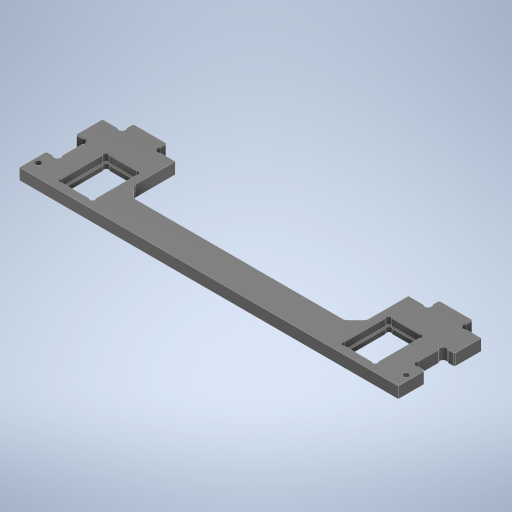
# Autodesk Inventor part: TorsoElectronicBoxUpperFrame
Saved by Autodesk Inventor 2024.2 (Build 282272000, 272)
## iProperties
Created: 2024-01-24
Part Number: TorsoElectronicBoxUpperFrame
Material: Acetal Resin, Black
Document SubType Name: Modeling
Designer: Masato Kubotera
Density: 1.425 g/cm^3
Appearance: Smooth - Black
Mass: 23.1569 g
Surface Area: 99.1055 cm^2
Volume: 16.2504 cm^3
Vendor: meviy
Author: Masato Kubotera
Autodesk Inventor part; units mm, degrees
ref_plane "YZ Plane" through (0, 0, 0) normal (1, 0, 0) x (0, 1, 0)
ref_plane "XZ Plane" through (0, 0, 0) normal (0, 1, 0) x (-1, 0, 0)
ref_plane "XY Plane" through (0, 0, 0) normal (0, 0, 1) x (1, 0, 0)
sketch "Sketch1" plane through (0, 0, 0) normal (0, 0, 1) x (1, 0, 0)
  line L0 (0, -84.5) -> (0, -75.75)
  line L1 (0, -75.75) -> (-5, -75.75)
  line L2 (-5, -75.75) -> (-5, -60.75)
  line L3 (-5, -60.75) -> (0, -60.75)
  line L4 (0, -60.75) -> (0, 60.75)
  line L5 (0, 0) -> (37, 0) construction
  line L6 (0, -84.5) -> (11.95, -84.5)
  line L7 (11.95, -84.5) -> (11.95, -79.5)
  line L8 (11.95, -79.5) -> (25.05, -79.5)
  line L9 (25.05, -79.5) -> (25.05, -84.5)
  line L10 (25.05, -84.5) -> (37, -84.5)
  line L11 (37, -84.5) -> (37, 84.5)
  line L12 (0, 84.5) -> (0, 75.75)
  line L13 (0, 75.75) -> (-5, 75.75)
  line L14 (-5, 75.75) -> (-5, 60.75)
  line L15 (-5, 60.75) -> (0, 60.75)
  line L16 (0, 84.5) -> (11.95, 84.5)
  line L17 (11.95, 84.5) -> (11.95, 79.5)
  line L18 (11.95, 79.5) -> (25.05, 79.5)
  line L19 (25.05, 79.5) -> (25.05, 84.5)
  line L20 (25.05, 84.5) -> (37, 84.5)
  arc A0 (14.0713, -79.5) -> (11.95, -81.6213) centre (13.0107, -80.5607) ccw
  line L21 (12, -84.5) -> (12, -79.5) construction
  line L22 (18.5, -79.5) -> (18.5, -84.5) construction
  line L23 (25, -84.5) -> (25, -79.5) construction
  arc A1 (0, -77.8713) -> (-2.1213, -75.75) centre (-1.0607, -76.8107) ccw
  line L24 (-5, -68.25) -> (0, -68.25) construction
  arc A2 (-2.1213, -60.75) -> (0, -58.6287) centre (-1.0607, -59.6893) ccw
  arc A3 (25.05, -81.6213) -> (22.9287, -79.5) centre (23.9893, -80.5607) ccw
  line L25 (18.5, -82) -> (31, -82) construction
  arc A4 (11.95, 81.6213) -> (14.0713, 79.5) centre (13.0107, 80.5607) ccw
  arc A5 (-2.1213, 75.75) -> (0, 77.8713) centre (-1.0607, 76.8107) ccw
  arc A6 (0, 58.6287) -> (-2.1213, 60.75) centre (-1.0607, 59.6893) ccw
  arc A7 (22.9287, 79.5) -> (25.05, 81.6213) centre (23.9893, 80.5607) ccw
  line L26 (0, -52) -> (23.5, -52)
  line L27 (23.5, -52) -> (23.5, 52)
  line L28 (23.5, 52) -> (0, 52)
  line L29 (23, 51.5) -> (23, -51.5) construction
  line L30 (32.5, -69.5) -> (13.3, -69.5) construction
  line L31 (13.3, -69.5) -> (13.3, -56.6) construction
  line L32 (13.3, -56.6) -> (32.5, -56.6) construction
  line L33 (32.5, -56.6) -> (32.5, -69.5) construction
  line L34 (32.5, -69.5) -> (13.3, -56.6) construction
  line L35 (13.3, -69.5) -> (32.5, -56.6) construction
  line L36 (12.35, -55.5) -> (33.45, -55.5) construction
  line L37 (33.45, -55.5) -> (33.45, -70.6) construction
  line L38 (33.45, -70.6) -> (12.35, -70.6) construction
  line L39 (12.35, -70.6) -> (12.35, -55.5) construction
  line L40 (12.35, -55.5) -> (33.45, -70.6) construction
  line L41 (33.45, -55.5) -> (12.35, -70.6) construction
  line L42 (13.7849, -55.45) -> (32.0151, -55.45)
  line L43 (33.5, -56.9349) -> (33.5, -69.1651)
  line L44 (33.5, -70.65) -> (12.3, -55.45) construction
  line L45 (12.3, -70.65) -> (33.5, -55.45) construction
  line L46 (32.55, -69.55) -> (13.25, -56.55) construction
  line L47 (13.25, -69.55) -> (32.55, -56.55) construction
  arc A8 (13.7849, -55.45) -> (12.3, -56.9349) centre (13.0425, -56.1925) ccw
  arc A9 (14.7349, -56.55) -> (13.25, -58.0349) centre (13.9925, -57.2925) ccw
  line L48 (12.3, -63.05) -> (33.5, -63.05) construction
  line L49 (22.9, -55.45) -> (22.9, -70.65) construction
  arc A10 (33.5, -56.9349) -> (32.0151, -55.45) centre (32.7575, -56.1925) ccw
  arc A11 (32.55, -58.0349) -> (31.0651, -56.55) centre (31.8075, -57.2925) ccw
  arc A12 (13.25, -68.0651) -> (14.7349, -69.55) centre (13.9925, -68.8075) ccw
  arc A13 (12.3, -69.1651) -> (13.7849, -70.65) centre (13.0425, -69.9075) ccw
  arc A14 (31.0651, -69.55) -> (32.55, -68.0651) centre (31.8075, -68.8075) ccw
  arc A15 (32.0151, -70.65) -> (33.5, -69.1651) centre (32.7575, -69.9075) ccw
  line L50 (14.7349, -56.55) -> (31.0651, -56.55)
  line L51 (32.55, -58.0349) -> (32.55, -68.0651)
  line L52 (12.3, -69.1651) -> (12.3, -56.9349)
  line L53 (13.25, -68.0651) -> (13.25, -58.0349)
  line L54 (31.0651, -69.55) -> (14.7349, -69.55)
  line L55 (32.0151, -70.65) -> (13.7849, -70.65)
  line L56 (13.3, 69.5) -> (13.3, 56.6) construction
  arc A16 (12.3, 56.9349) -> (13.7849, 55.45) centre (13.0425, 56.1925) ccw
  arc A17 (13.7849, 70.65) -> (12.3, 69.1651) centre (13.0425, 69.9075) ccw
  line L57 (14.7349, 56.55) -> (31.0651, 56.55)
  arc A18 (32.0151, 55.45) -> (33.5, 56.9349) centre (32.7575, 56.1925) ccw
  arc A19 (31.0651, 56.55) -> (32.55, 58.0349) centre (31.8075, 57.2925) ccw
  line L58 (32.55, 58.0349) -> (32.55, 68.0651)
  line L59 (33.5, 56.9349) -> (33.5, 69.1651)
  line L60 (31.0651, 69.55) -> (14.7349, 69.55)
  arc A20 (32.55, 68.0651) -> (31.0651, 69.55) centre (31.8075, 68.8075) ccw
  arc A21 (33.5, 69.1651) -> (32.0151, 70.65) centre (32.7575, 69.9075) ccw
  line L61 (32.0151, 70.65) -> (13.7849, 70.65)
  line L62 (22.9, 55.45) -> (22.9, 70.65) construction
  line L63 (13.7849, 55.45) -> (32.0151, 55.45)
  line L64 (32.5, 69.5) -> (13.3, 69.5) construction
  line L65 (13.3, 56.6) -> (32.5, 56.6) construction
  line L66 (32.5, 56.6) -> (32.5, 69.5) construction
  line L67 (32.5, 69.5) -> (13.3, 56.6) construction
  line L68 (13.3, 69.5) -> (32.5, 56.6) construction
  line L69 (12.35, 55.5) -> (33.45, 55.5) construction
  line L70 (33.45, 55.5) -> (33.45, 70.6) construction
  line L71 (33.45, 70.6) -> (12.35, 70.6) construction
  line L72 (12.35, 70.6) -> (12.35, 55.5) construction
  line L73 (12.35, 55.5) -> (33.45, 70.6) construction
  line L74 (33.45, 55.5) -> (12.35, 70.6) construction
  line L75 (12.3, 70.65) -> (33.5, 55.45) construction
  line L76 (32.55, 69.55) -> (13.25, 56.55) construction
  line L77 (13.25, 69.55) -> (32.55, 56.55) construction
  arc A22 (13.25, 58.0349) -> (14.7349, 56.55) centre (13.9925, 57.2925) ccw
  line L78 (12.3, 63.05) -> (33.5, 63.05) construction
  arc A23 (14.7349, 69.55) -> (13.25, 68.0651) centre (13.9925, 68.8075) ccw
  line L79 (13.25, 68.0651) -> (13.25, 58.0349)
  line L80 (12.3, 69.1651) -> (12.3, 56.9349)
  line L81 (33.5, 70.65) -> (12.3, 55.45) construction
  line L82 (23, -51.5) -> (0, -51.5) construction
  line L83 (23, 51.5) -> (0, 51.5) construction
  point P0 (31, 82)
  point P1 (22.9287, -79.5)
  point P2 (25.05, -81.6213)
  point P3 (25.05, 81.6213)
  point P4 (22.9287, 79.5)
  point P5 (14.0713, 79.5)
  point P6 (11.95, 81.6213)
  point P7 (0, 77.8713)
  point P8 (-2.1213, 75.75)
  point P9 (-2.1213, 60.75)
  point P10 (0, 58.6287)
  point P11 (0, -58.6287)
  point P12 (-2.1213, -60.75)
  point P13 (22.9, -63.05)
  point P14 (22.9, -63.05)
  point P15 (22.9, 63.05)
  point P16 (22.9, 63.05)
  point P17 (25.05, 79.5)
  point P18 (0, 60.75)
  point P19 (25.05, 79.5)
  point P20 (0, 75.75)
  point P21 (0, 60.75)
  point P22 (11.95, 79.5)
  point P23 (0, 75.75)
  point P24 (11.95, 79.5)
  point P25 (0, -60.75)
  point P26 (25.05, -79.5)
  point P27 (0, -60.75)
  point P28 (0, -52)
  dimension "d0" = 5
  dimension "d1" = 5
  dimension "d2" = 1.5
  dimension "d4" = 15
  dimension "d5" = 0.05
  dimension "d6" = 12
  dimension "d7" = 169
  dimension "d8" = 37
  dimension "d9" = 6
  dimension "d22" = 23
  dimension "d28" = 19.2
  dimension "d29" = 12.9
  dimension "d30" = 21.1
  dimension "d31" = 15.1
  dimension "d32" = 0.05
  dimension "d33" = 1.05
  dimension "d34" = 1.05
  dimension "d35" = 0.05
  dimension "d36" = 0.05
  dimension "d37" = 0.05
  dimension "d44" = 3.5
  dimension "d46" = 3.5
  dimension "d52" = 13.5
  dimension "d53" = 0.5
  dimension "d54" = 103
  dimension "d55" = 0.5
  dimension "d60" = 22.5
  constraints: 168 end point, 96 symmetric about line, 58 point on circle, 29 midpoint, 27 point on line, 24 centre point, 13 horizontal, 9 parallel, 7 vertical, 6 perpendicular, 1 equal radius, 23 other
  measures "d0" distance of L0.end L1.end
  measures "d1" distance of L7.end L6.end
  measures "d2" radius of A0
  measures "d4" distance of L1.end L2.end
  measures "d5" distance between parallel lines of L21 L7
  measures "d6" distance between parallel lines of L21 L0
  measures "d7" distance of L10.end L11.end
  measures "d8" distance of L10.end L0.start
  measures "d9" distance from line of L25.end L23
  measures "d22" distance between parallel lines of L4 L29
  measures "d28" distance of L31.end L32.end
  measures "d29" distance of L31.start L31.end
  measures "d30" distance of L37.end L38.end
  measures "d31" distance of L36.end L37.end
  measures "d32" distance between parallel lines of L42 L36
  measures "d33" radius of A8
  measures "d34" radius of A9
  measures "d35" distance between parallel lines of L50 L32
  measures "d36" distance between parallel lines of L52 L39
  measures "d37" distance between parallel lines of L53 L31
  measures "d44" distance between parallel lines of L11 L43
  measures "d46" distance between parallel lines of L26 L36
  measures "d52" distance between parallel lines of L11 L27
  measures "d53" distance between parallel lines of L27 L29
  measures "d54" distance of L29.start L29.end
  measures "d55" distance between parallel lines of L82 L26
  measures "d60" diameter of L8 L24
extrude "Extrusion1" add sketch "Sketch1" against normal blind 5 contours L0 A1 L1 L2 L3 A2 L4 L26 L27 L28 A6 L15 L14 L13 A5 L12 L16 L17 A4 L18 A7 L19 L20 L11 L10 L9 A3 L8 A0 L7 L6 | L42 A10 L43 A15 L55 A13 L52 A8 | L80 A17 L61 A21 L59 A18 L63 A16
extrude "Extrusion2" cut sketch "Sketch1" against normal blind 3 contours L42 A10 L43 A15 L55 A13 L52 A8 | L80 A17 L61 A21 L59 A18 L63 A16
hole "Phi2.5" at (31, -82, 0) at (31, 82, 0) direction (0, 0, -1) diameter 2.5 end through all
chamfer "C0.5" distance 0.5 angle 45 8 edges at (-5, -60.75, -2.5) (-5, -75.75, -2.5) (-5, 75.75, -2.5) (-5, 60.75, -2.5) (11.95, -84.5, -2.5) (25.05, -84.5, -2.5) (11.95, 84.5, -2.5) (25.05, 84.5, -2.5)
chamfer "C5" distance 5 angle 45 2 edges at (23.5, -52, -2.5) (23.5, 52, -2.5)
fillet "R2" radius 2 4 edges at (18.5, -52, -2.5) (23.5, -47, -2.5) (23.5, 47, -2.5) (18.5, 52, -2.5)
ref_plane "Work Plane1" through (14.7349, -63.05, -5) normal (0, -1, 0) x (1, 0, 0)
ref_plane "Work Plane2" through (22.9, -68.0651, -5) normal (1, 0, 0) x (0, 0, -1)
ref_plane "Work Plane3" through (14.7349, 63.05, -5) normal (0, 1, 0) x (1, 0, 0)
equation "\"d34\" = d33"
equation "\"d35\" = d32"
equation "\"d36\" = d32"
equation "\"d37\" = d32"
equation "\"d46\" = d44"
body "Solid1"
